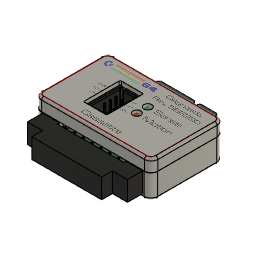
Diag_CP_PCB_v1 v16 (Autodesk Fusion 360 design; units mm, degrees)
Autodesk Fusion 360 part; units mm, degrees
note: some values were not read from the file. Chosen so that the rebuilt part matches the saved one: which bodies a step acts on; which face or edge a step refers to.
sketch "dxf import" plane through (0, 0, 0) normal (0, 0, 1) x (1, 0, 0) in component "PCB"
  line L0 (29, 0) -> (1, 0)
  line L1 (0.7, 29) -> (0, 29)
  line L2 (0, 1) -> (0, 29)
  arc A0 (0.7, 29) -> (1.5, 29.8) centre (0.7, 29.8) ccw
  arc A1 (28.5, 30.8) -> (29.3, 30) centre (29.3, 30.8) ccw
  line L3 (30, 30) -> (30, 29)
  line L4 (29.3, 30) -> (30, 30)
  line L5 (30, 29) -> (30, 1)
  line L6 (1.5, 31) -> (1.5, 29.8)
  line L7 (26, 43) -> (27.5, 43)
  line L8 (27.5, 43) -> (28.5, 42)
  line L9 (28.5, 42) -> (28.5, 31)
  line L10 (1.5, 42) -> (1.5, 31)
  arc A2 (29, 0) -> (30, 1) centre (29, 1) ccw
  line L11 (18.16, 33) -> (18.16, 42.2)
  arc A3 (20.56, 43) -> (19.76, 42.2) centre (20.56, 42.2) ccw
  line L12 (19.76, 42.2) -> (19.76, 33)
  line L13 (28.5, 31) -> (28.5, 30.8)
  arc A4 (0, 1) -> (1, 0) centre (1, 1) ccw
  line L14 (17.36, 43) -> (2.5, 43)
  arc A5 (18.16, 33) -> (18.96, 32.2) centre (18.96, 33) ccw
  line L15 (2.5, 43) -> (1.5, 42)
  line L16 (26, 43) -> (20.56, 43)
  arc A6 (18.96, 32.2) -> (19.76, 33) centre (18.96, 33) ccw
  arc A7 (18.16, 42.2) -> (17.36, 43) centre (17.36, 42.2) ccw
  line L17 (14.72, 0) -> (14.72, -1)
  line L18 (22.64, 0) -> (22.64, -1)
  line L19 (15.95, 0.1) -> (15.95, -1)
  line L20 (17.95, 0.1) -> (17.95, -1)
  line L21 (21.91, 0.1) -> (21.91, -1)
  line L22 (27.1, 0) -> (26.6, 0)
  line L23 (19.18, 0) -> (18.68, 0)
  line L24 (15.22, 0) -> (14.72, 0)
  circle A8 centre (25.4, 25.4) radius 1.7463
  line L25 (23.14, 0) -> (22.64, 0)
  line L26 (10.76, 0) -> (10.76, -1)
  line L27 (25.87, 0.1) -> (25.87, -1)
  line L28 (15.22, -1) -> (15.22, 0)
  circle A9 centre (25.4, 25.4) radius 3.1789
  line L29 (11.26, -1) -> (11.26, 0)
  line L30 (23.14, -1) -> (23.14, 0)
  line L31 (18.68, 0) -> (18.68, -1)
  line L32 (26.6, 0) -> (26.6, -1)
  line L33 (19.18, -1) -> (19.18, 0)
  line L34 (13.99, 0.1) -> (13.99, -1)
  line L35 (23.87, 0.1) -> (23.87, -1)
  line L36 (19.91, 0.1) -> (19.91, -1)
  line L37 (27.1, -1) -> (27.1, 0)
  line L38 (11.99, 0.1) -> (11.99, -1)
  line L39 (11.26, 0) -> (10.76, 0)
  line L40 (-4.15, -8.7333) -> (-4.15, -11.6)
  line L41 (0.05, -1) -> (0.05, 0)
  line L42 (34.09, -11.6) -> (34.09, -8.7333)
  line L43 (34.09, -3.6853) -> (34.09, -3.548)
  line L44 (-5.85, -6.8) -> (-5.85, -5.2)
  line L45 (10.03, 0.1) -> (10.03, -1)
  line L46 (37.34, -6.8) -> (35.79, -6.8)
  line L47 (34.09, -8.052) -> (34.09, -7.9147)
  line L48 (-5.85, -1.6) -> (-5.85, 0)
  line L49 (-4.15, 0) -> (-4.15, -2.8667)
  line L50 (-5.85, -6.8) -> (-7.4, -6.8)
  line L51 (35.79, 0) -> (34.09, 0)
  line L52 (8.03, 0.1) -> (8.03, -1)
  line L53 (37.34, 0) -> (35.79, 0)
  line L54 (3.34, -1) -> (3.34, 0)
  line L55 (34.09, -7.2333) -> (34.09, -4.3667)
  line L56 (-2.45, -6.8) -> (-5.85, -6.8)
  line L57 (-5.85, -4.2) -> (-5.85, -2.6)
  line L58 (-2.45, 0) -> (-4.15, 0)
  line L59 (32.39, -6.8) -> (30.59, -6.8)
  line L60 (0.05, 0) -> (-2.45, 0)
  line L61 (34.09, -2.8667) -> (34.09, 0)
  line L62 (-2.45, -6.8) -> (-2.45, -5.2)
  line L63 (-5.85, 0) -> (-7.4, 0)
  line L64 (-2.45, -1.6) -> (-2.45, 0)
  line L65 (-2.45, -4.2) -> (-2.45, -2.6)
  line L66 (-0.65, -11.6) -> (-0.65, -6.8)
  line L67 (32.39, 0) -> (29.89, 0)
  line L68 (-7.4, 0) -> (-7.4, -6.8)
  line L69 (30.59, -11.6) -> (-0.65, -11.6)
  line L70 (7.3, 0) -> (6.8, 0)
  line L71 (-0.65, -6.8) -> (-2.45, -6.8)
  line L72 (1.4287, 6.0325) -> (2.6987, 6.0325)
  line L73 (3.3338, 5.3975) -> (3.3338, 4.1275)
  line L74 (2.6987, 6.0325) -> (3.3338, 5.3975)
  line L75 (30.59, -6.8) -> (30.59, -11.6)
  line L76 (37.34, 0) -> (37.34, -6.8)
  line L77 (16.0338, 11.43) -> (16.0338, 8.89)
  line L78 (23.6538, 11.43) -> (16.0338, 11.43)
  line L79 (6.8, 0) -> (6.8, -1)
  line L80 (0.7938, 4.1275) -> (0.7938, 5.3975)
  line L81 (0.7938, 5.3975) -> (1.4287, 6.0325)
  line L82 (16.8275, 24.4475) -> (16.8275, 26.9875)
  line L83 (4.07, 0.1) -> (4.07, -1)
  line L84 (34.09, 0) -> (32.39, 0)
  line L85 (6.07, 0.1) -> (6.07, -1)
  line L86 (1.4287, 3.4925) -> (2.6987, 3.4925)
  line L87 (-4.15, -7.9147) -> (-4.15, -8.052)
  line L88 (-4.15, -3.548) -> (-4.15, -3.6853)
  line L89 (2.6987, 3.4925) -> (3.3338, 4.1275)
  line L90 (0.7938, 4.1275) -> (1.4287, 3.4925)
  line L91 (16.0338, 10.16) -> (15.2718, 10.16)
  line L92 (7.3, -1) -> (7.3, 0)
  line L93 (3.34, 0) -> (2.84, 0)
  line L94 (-4.15, 0) -> (-5.85, 0)
  arc A10 (25.5672, 18.0901) -> (21.3677, 19.3984) centre (23.0187, 17.3038) ccw
  line L95 (-4.15, -4.3667) -> (-4.15, -7.2333)
  line L96 (15.875, 22.3838) -> (13.335, 22.3838)
  line L97 (9.2075, 24.4475) -> (16.8275, 24.4475)
  line L98 (29.89, 0) -> (29.89, -1)
  line L99 (15.875, 14.7637) -> (15.875, 22.3838)
  line L100 (35.79, -4.2) -> (35.79, -2.6)
  line L101 (23.6538, 10.16) -> (24.4158, 10.16)
  line L102 (16.8275, 25.7175) -> (17.5895, 25.7175)
  line L103 (35.79, -6.8) -> (32.39, -6.8)
  line L104 (29.89, -1) -> (0.05, -1)
  line L105 (35.79, -6.8) -> (35.79, -5.2)
  line L106 (2.84, 0) -> (2.84, -1)
  arc A11 (17.8675, 14.44) -> (20.8675, 14.44) centre (19.3675, 15.24) ccw
  line L107 (14.605, 14.7637) -> (14.605, 14.0018)
  line L108 (21.3678, 19.3987) -> (21.3678, 15.2088)
  line L109 (16.0338, 8.89) -> (23.6538, 8.89)
  line L110 (13.335, 14.7637) -> (15.875, 14.7637)
  arc A12 (20.8675, 16.04) -> (17.8675, 16.04) centre (19.3675, 15.24) ccw
  line L111 (13.335, 22.3838) -> (13.335, 14.7637)
  arc A13 (21.3677, 15.2087) -> (25.5672, 16.5169) centre (23.0187, 17.3032) ccw
  line L112 (22.7647, 19.9588) -> (22.7647, 19.5578)
  line L113 (16.8275, 26.9875) -> (9.2075, 26.9875)
  line L114 (9.2075, 25.7175) -> (8.4455, 25.7175)
  arc A14 (20.8675, 16.04) -> (17.8675, 16.04) centre (19.3675, 15.24) ccw
  line L115 (22.7647, 15.0498) -> (22.7647, 14.6488)
  arc A15 (17.8675, 14.44) -> (20.8675, 14.44) centre (19.3675, 15.24) ccw
  line L116 (23.6538, 8.89) -> (23.6538, 11.43)
  line L117 (14.605, 22.3838) -> (14.605, 23.1457)
  line L118 (22.7647, 17.5898) -> (22.7647, 17.0177)
  line L119 (9.2075, 26.9875) -> (9.2075, 24.4475)
  line L120 (4.33, 9.1737) -> (4.8062, 9.65)
  arc A16 (3.5362, 10.92) -> (3.5362, 9.65) centre (3.5362, 10.285) ccw
  line L121 (11.95, 9.1737) -> (11.4738, 9.65)
  arc A17 (3.5362, 16.4763) -> (3.5362, 15.3651) centre (3.5362, 15.9207) ccw
  line L122 (6.3937, 23.62) -> (12.7438, 23.62)
  line L123 (4.33, 9.1737) -> (4.965, 9.1737)
  arc A18 (3.5362, 22.35) -> (3.5362, 21.08) centre (3.5362, 21.715) ccw
  line L124 (4.33, 9.1737) -> (4.33, 22.8263)
  line L125 (11.4738, 22.35) -> (11.4738, 17.27)
  line L126 (6.3937, 22.35) -> (11.4738, 22.35)
  line L127 (12.7438, 8.38) -> (6.3937, 8.38)
  line L128 (6.3937, 9.65) -> (6.3937, 9.1737)
  line L129 (4.965, 9.1737) -> (4.965, 8.38)
  line L130 (4.965, 9.65) -> (4.965, 9.1737)
  line L131 (6.3937, 9.1737) -> (11.95, 9.1737)
  line L132 (3.5362, 23.62) -> (4.965, 23.62)
  line L133 (11.95, 14.73) -> (11.95, 9.1737)
  line L134 (4.965, 22.8263) -> (4.33, 22.8263)
  line L135 (6.3937, 9.65) -> (4.965, 9.65)
  line L136 (12.7438, 14.73) -> (12.7438, 8.38)
  line L137 (4.8062, 22.35) -> (4.965, 22.35)
  line L138 (4.965, 22.35) -> (4.965, 22.8263)
  line L139 (3.5362, 8.38) -> (3.5362, 23.62)
  line L140 (6.3937, 8.38) -> (4.965, 8.38)
  line L141 (4.8062, 9.65) -> (4.8062, 22.35)
  line L142 (11.4738, 14.73) -> (11.4738, 9.65)
  line L143 (6.3937, 9.1737) -> (6.3937, 8.38)
  line L144 (4.965, 22.35) -> (6.3937, 22.35)
  line L145 (11.4738, 14.73) -> (11.95, 14.73)
  line L146 (11.4738, 17.27) -> (11.4738, 14.73)
  line L147 (11.95, 14.73) -> (12.7438, 14.73)
  line L148 (4.965, 22.8263) -> (4.965, 23.62)
  line L149 (4.965, 8.38) -> (3.5362, 8.38)
  line L150 (11.4738, 17.27) -> (11.95, 17.27)
  line L151 (4.965, 23.62) -> (6.3937, 23.62)
  line L152 (11.95, 17.27) -> (11.95, 22.8263)
  line L153 (6.3937, 22.35) -> (6.3937, 22.8263)
  line L154 (6.3937, 22.8263) -> (6.3937, 23.62)
  line L155 (6.3937, 22.8263) -> (11.95, 22.8263)
  line L156 (12.7438, 23.62) -> (12.7438, 17.27)
  line L157 (12.7438, 17.27) -> (12.7438, 14.73)
  line L158 (11.95, 17.27) -> (12.7438, 17.27)
  line L159 (11.4738, 9.65) -> (6.3937, 9.65)
  line L160 (4.965, 9.65) -> (4.8062, 9.65)
  line L161 (35.79, -1.6) -> (35.79, 0)
  line L162 (32.39, -1.6) -> (32.39, 0)
  line L163 (4.8062, 22.35) -> (4.33, 22.8263)
  line L164 (32.39, -4.2) -> (32.39, -2.6)
  line L165 (32.39, -6.8) -> (32.39, -5.2)
  line L166 (11.4738, 22.35) -> (11.95, 22.8263)
  line L167 (11.99, 0.1) -> (11.99, 4)
  line L168 (13.99, 0.1) -> (13.99, 4)
  arc A19 (13.99, 4) -> (11.99, 4) centre (12.99, 4) ccw
  arc A20 (25.87, 4) -> (23.87, 4) centre (24.87, 4) ccw
  line L169 (23.87, 0.1) -> (23.87, 4)
  arc A21 (16.45, 2) -> (17.45, 2) centre (16.95, 2) ccw
  arc A22 (17.45, 3) -> (16.45, 3) centre (16.95, 3) ccw
  arc A23 (20.41, 2) -> (21.41, 2) centre (20.91, 2) ccw
  line L170 (19.91, 0.1) -> (19.91, 4)
  line L171 (13.49, 3) -> (13.49, 2)
  line L172 (12.49, 3) -> (12.49, 2)
  arc A24 (13.49, 3) -> (12.49, 3) centre (12.99, 3) ccw
  arc A25 (12.49, 2) -> (13.49, 2) centre (12.99, 2) ccw
  line L173 (25.37, 3) -> (25.37, 2)
  line L174 (20.41, 3) -> (20.41, 2)
  line L175 (17.45, 3) -> (17.45, 2)
  arc A26 (21.41, 3) -> (20.41, 3) centre (20.91, 3) ccw
  arc A27 (25.37, 3) -> (24.37, 3) centre (24.87, 3) ccw
  line L176 (17.95, 0.1) -> (17.95, 4)
  line L177 (16.45, 3) -> (16.45, 2)
  line L178 (21.41, 3) -> (21.41, 2)
  line L179 (5.57, 3) -> (5.57, 2)
  arc A28 (9.53, 3) -> (8.53, 3) centre (9.03, 3) ccw
  arc A29 (8.53, 2) -> (9.53, 2) centre (9.03, 2) ccw
  line L180 (6.616, 13.714) -> (6.616, 13.206)
  line L181 (9.664, 13.206) -> (9.664, 13.714)
  line L182 (7.124, 18.794) -> (6.616, 18.794)
  line L183 (6.616, 15.746) -> (7.124, 15.746)
  line L184 (7.124, 13.206) -> (7.124, 13.714)
  line L185 (24.37, 3) -> (24.37, 2)
  line L186 (7.124, 16.254) -> (6.616, 16.254)
  line L187 (6.616, 16.254) -> (6.616, 15.746)
  line L188 (9.156, 15.746) -> (9.664, 15.746)
  line L189 (1.8098, 5.0165) -> (1.8098, 4.5085)
  line L190 (8.53, 3) -> (8.53, 2)
  line L191 (2.3178, 5.0165) -> (1.8098, 5.0165)
  line L192 (9.156, 13.714) -> (9.156, 13.206)
  arc A30 (5.57, 3) -> (4.57, 3) centre (5.07, 3) ccw
  line L193 (4.07, 0.1) -> (4.07, 4)
  line L194 (10.03, 0.1) -> (10.03, 4)
  arc A31 (17.95, 4) -> (15.95, 4) centre (16.95, 4) ccw
  line L195 (4.57, 3) -> (4.57, 2)
  line L196 (15.95, 0.1) -> (15.95, 4)
  arc A32 (10.03, 4) -> (8.03, 4) centre (9.03, 4) ccw
  line L197 (7.124, 15.746) -> (7.124, 16.254)
  line L198 (6.616, 18.286) -> (7.124, 18.286)
  line L199 (9.664, 13.714) -> (9.156, 13.714)
  line L200 (9.156, 18.286) -> (9.664, 18.286)
  line L201 (7.124, 13.714) -> (6.616, 13.714)
  line L202 (9.156, 18.794) -> (9.156, 18.286)
  line L203 (7.124, 18.286) -> (7.124, 18.794)
  line L204 (21.91, 0.1) -> (21.91, 4)
  arc A33 (24.37, 2) -> (25.37, 2) centre (24.87, 2) ccw
  line L205 (9.53, 3) -> (9.53, 2)
  line L206 (9.156, 13.206) -> (9.664, 13.206)
  line L207 (9.664, 18.794) -> (9.156, 18.794)
  line L208 (2.3178, 4.5085) -> (2.3178, 5.0165)
  line L209 (9.156, 16.254) -> (9.156, 15.746)
  arc A34 (6.07, 4) -> (4.07, 4) centre (5.07, 4) ccw
  arc A35 (4.57, 2) -> (5.57, 2) centre (5.07, 2) ccw
  line L210 (6.07, 0.1) -> (6.07, 4)
  line L211 (9.664, 15.746) -> (9.664, 16.254)
  line L212 (6.616, 18.794) -> (6.616, 18.286)
  arc A36 (21.91, 4) -> (19.91, 4) centre (20.91, 4) ccw
  line L213 (8.03, 0.1) -> (8.03, 4)
  line L214 (9.664, 16.254) -> (9.156, 16.254)
  line L215 (6.616, 13.206) -> (7.124, 13.206)
  line L216 (20.8675, 16.04) -> (20.8675, 14.44)
  circle A37 centre (19.3675, 15.24) radius 1.5
  arc A38 (17.8675, 16.04) -> (17.8675, 14.44) centre (19.3675, 15.24) ccw
  circle A39 centre (19.3675, 20.1613) radius 1.5
  line L217 (9.664, 18.286) -> (9.664, 18.794)
  line L218 (1.8098, 4.5085) -> (2.3178, 4.5085)
  arc A40 (25.5673, 16.5175) -> (25.5673, 18.0901) centre (23.0188, 17.3038) ccw
  line L219 (22.7647, 19.5578) -> (22.7647, 17.5898)
  line L220 (22.7647, 17.0177) -> (22.7647, 15.0498)
  line L221 (25.87, 0.1) -> (25.87, 4)
  line L222 (20.8588, 20.9774) -> (20.876, 19.3775)
  arc A41 (20.8588, 20.9774) -> (20.876, 19.3775) centre (19.3675, 20.1613) ccw
  line L223 (1.8098, 5.0165) -> (2.3178, 4.5085) construction
  constraint tangent A39 L222
extrude "Extrude1" add sketch "dxf import" against normal blind 1.6 contours L0 L1 L2 A0 A1 L3 L4 L5 L6 L7 L8 L9 L10 A2 L11 A3 L12 L13 A4 L14 A5 L15 L16 A6 A7 L19 L20 L21 L22 L23 L24 L25 L27 L34 L35 L36 L38 L39 L45 L52 L70 L83 L85 L93 L167 L168 A19 A20 L169 L170 L176 L193 L194 A31 L196 A32 L204 A34 L210 A36 L213 L221 | L0 L27 L35 A20 L169 L221 | L0 L21 L36 L170 L204 A36 | L0 L19 L20 L176 A31 L196 | L0 L34 L38 L167 L168 A19 | L0 L45 L52 L194 A32 L213 | L0 L83 L85 L193 A34 L210 | A9 | L72 L73 L74 L80 L81 L86 L89 L90 | L77 L78 L109 L116 | L82 L97 L113 L119 | A10 A13 L112 L115 L118 A40 L219 L220 | A10 L108 A13 L112 L115 L118 L219 L220 | L96 L99 L110 L111 | A37 | A11 A12 A14 A15 L216 A38 | L120 L124 L141 L163 | L120 L123 L130 L160 | L123 L124 L129 L132 L134 L139 L148 L149 | L125 L126 L135 L137 L141 L142 L144 L146 L159 L160 | L128 L129 L130 L135 L140 L143 | L134 L137 L138 L163 | L138 L144 L148 L151 L153 L154 | L121 L128 L131 L159 | L127 L131 L133 L136 L143 L147 | L126 L153 L155 L166 | L121 L133 L142 L145 | A16 L139 | L122 L152 L154 L155 L156 L158 | L125 L150 L152 L166 | L145 L146 L147 L150 L157 L158 | A18 L139 | A17 L139 | A21 A22 L175 L177 | A23 L174 A26 L178 | L171 L172 A24 A25 | L173 A27 L185 A33 | L179 A30 L195 A35 | A28 A29 L190 L205 | L180 L184 L201 L215 | L181 L192 L199 L206 | L182 L198 L203 L212 | L183 L186 L187 L197 | L188 L209 L211 L214 | L189 L191 L208 L218 | L200 L202 L207 L217 | A39 | L222 A41 makes body 1 in component "PCB"
extrude "Extrude2" add sketch "dxf import" along normal blind 2.2 contours L125 L126 L135 L137 L141 L142 L144 L146 L159 L160 | L128 L129 L130 L135 L140 L143 | L138 L144 L148 L151 L153 L154 | L145 L146 L147 L150 L157 L158 bodies 1 in component "PCB"
extrude "Extrude3" add sketch "dxf import" along normal blind 8.5 contours L180 L184 L201 L215 | L181 L192 L199 L206 | L182 L198 L203 L212 | L183 L186 L187 L197 | L188 L209 L211 L214 | L200 L202 L207 L217 bodies 1 in component "PCB"
extrude "Extrude4" add sketch "dxf import" along normal blind 8.8 contours L120 L124 L141 L163 | L120 L123 L130 L160 | L123 L124 L129 L132 L134 L139 L148 L149 | L134 L137 L138 L163 | L121 L128 L131 L159 | L127 L131 L133 L136 L143 L147 | L126 L153 L155 L166 | L121 L133 L142 L145 | L122 L152 L154 L155 L156 L158 | L125 L150 L152 L166 bodies 1 in component "PCB"
chamfer "Chamfer1" distance 0.5 angle 45 7 edges at (4.8062, 16, 8.8) (4.8856, 9.65, 8.8) (4.8856, 22.35, 8.8) (8.9337, 9.65, 8.8) (11.4738, 12.19, 8.8) (11.4738, 19.81, 8.8) (8.9337, 22.35, 8.8) on bodies 1 in component "PCB"
extrude "Extrude5" add sketch "dxf import" along normal blind 4.4 from surface at 5.5 separate body contours A37 | A39 makes body 2 at (17.875, 20.0119, 8.4333) makes body 3 at (20.8656, 15.1652, 8.4333) in component "PCB"
extrude "Extrude6" add sketch "dxf import" along normal blind 1 from surface at 5.5 contours A11 A12 A14 A15 L216 A38 bodies 3 in component "PCB"
extrude "Extrude7" add sketch "dxf import" along normal blind 1 from surface at 5.5 contours L222 A41 bodies 2 in component "PCB"
fillet "Fillet1" radius 1.45 2 edges at (17.969, 19.6189, 9.9) (17.969, 14.6976, 9.9) on bodies 2 3 in component "PCB"
extrude "Extrude8" add sketch "dxf import" along normal blind 8.8 from surface at -4.6 separate body contours L0 L22 L32 L37 L104 | L41 L46 L50 L51 L53 L56 L58 L59 L60 L63 L66 L67 L68 L69 L71 L75 L76 L84 L94 L98 L103 L104 | L0 L18 L25 L30 L104 | L0 L23 L31 L33 L104 | L0 L17 L24 L28 L104 | L0 L26 L29 L39 L104 | L0 L70 L79 L92 L104 | L0 L54 L93 L104 L106 makes body 4 in component "PCB"
extrude "Extrude9" add sketch "dxf import" against normal blind 0.5 from surface at -1.6 contours L0 L27 L35 L104 | L0 L27 L35 A20 L169 L221 | L0 L21 L36 L104 | L0 L21 L36 L170 L204 A36 | L0 L19 L20 L104 | L0 L19 L20 L176 A31 L196 | L0 L34 L38 L104 | L0 L34 L38 L167 L168 A19 | L0 L45 L52 L104 | L0 L45 L52 L194 A32 L213 | L0 L83 L85 L104 | L0 L83 L85 L193 A34 L210 bodies 1 4 in component "PCB"
combine "Combine1" operation add target body 1 tool bodies 2 3 makes body 5 at (17.875, 20.0119, 7.8) makes body 6 at (20.86, 15.0906, 7.15) in component "PCB"
combine "Combine2" operation add target body 1 tool bodies 5 6 makes body 7 at (17.875, 20.0119, 7.8) makes body 8 at (20.86, 15.0906, 7.15) in component "PCB"
ref_plane "WorkPlane1" through (0, 0, -4.4) normal (0, 0, 1) x (1, 0, 0) in component "diag cp bottom shell"
sketch "bottom shell" plane through (0, 0, -4.4) normal (0, 0, 1) x (1, 0, 0) in component "diag cp bottom shell"
  line L0 (30, 30) -> (30, 1) construction
  line L1 (0, 1) -> (0, 29) construction
  line L2 (2.84, 0) -> (1, 0) construction
  circle A0 centre (25.4, 25.4) radius 1.7463 construction
  line L3 (-11, 3) -> (-11, 29.5)
  line L4 (-8, 32.5) -> (38, 32.5)
  line L5 (38, 0) -> (-8, 0)
  line L6 (41, 29.5) -> (41, 3)
  arc A1 (-8, 32.5) -> (-11, 29.5) centre (-8, 29.5) ccw
  arc A2 (41, 29.5) -> (38, 32.5) centre (38, 29.5) ccw
  arc A3 (38, 0) -> (41, 3) centre (38, 3) ccw
  arc A4 (-11, 3) -> (-8, 0) centre (-8, 3) ccw
  circle A5 centre (25.4, 25.4) radius 1.75
  circle A6 centre (25.4, 25.4) radius 3
  circle A7 centre (25.4, 25.4) radius 4.25
  arc A8 (39, 29.5) -> (38, 30.5) centre (38, 29.5) ccw
  line L7 (-8, 30.5) -> (38, 30.5)
  arc A9 (-8, 30.5) -> (-9, 29.5) centre (-8, 29.5) ccw
  line L8 (-9, 3) -> (-9, 29.5)
  arc A10 (-9, 3) -> (-8, 2) centre (-8, 3) ccw
  line L9 (38, 2) -> (-8, 2)
  arc A11 (38, 2) -> (39, 3) centre (38, 3) ccw
  line L10 (39, 29.5) -> (39, 3)
  arc A12 (39.8, 29.5) -> (38, 31.3) centre (38, 29.5) ccw
  arc A13 (-8, 31.3) -> (-9.8, 29.5) centre (-8, 29.5) ccw
  line L11 (-9.8, 3) -> (-9.8, 29.5)
  arc A14 (-9.8, 3) -> (-8, 1.2) centre (-8, 3) ccw
  arc A15 (38, 1.2) -> (39.8, 3) centre (38, 3) ccw
  line L12 (39.8, 29.5) -> (39.8, 3)
  line L13 (30.3, 2) -> (30.3, 0)
  line L14 (-0.3, 2) -> (-0.3, 0)
  line L15 (1.5, 42) -> (1.5, 29.8) construction
  line L16 (28.5, 42) -> (28.5, 30.8) construction
  line L17 (28.8, 32.5) -> (28.8, 30.5)
  line L18 (1.2, 32.5) -> (1.2, 30.5)
  line L19 (-8, 31.3) -> (1.5, 31.3)
  line L20 (28.5, 31.3) -> (38, 31.3)
  line L21 (38, 1.2) -> (30, 1.2)
  line L22 (0, 1.2) -> (-8, 1.2)
  circle A16 centre (-4.5, 6.5) radius 1.75
  circle A17 centre (34.5, 6.5) radius 1.75
  circle A18 centre (-4.5, 6.5) radius 4
  circle A19 centre (34.5, 6.5) radius 4
  circle A20 centre (-4.5, 6.5) radius 3
  circle A21 centre (34.5, 6.5) radius 3
  line L23 (25.4, 25.4) -> (-9, 25.4) construction
  line L24 (-2, 26.4) -> (2, 26.4)
  line L25 (2, 26.4) -> (2, 24.4)
  line L26 (2, 24.4) -> (-2, 24.4)
  line L27 (-2, 24.4) -> (-2, 26.4)
  line L28 (-0.3, 26.4) -> (-0.3, 24.4)
  point P0 (-11, 0)
  point P1 (-11, 32.5)
  point P2 (41, 32.5)
  dimension "d54" = 3
  dimension "d55" = 11
  dimension "d56" = 32.5
  dimension "d57" = 52
  dimension "d59" = 3.5
  dimension "d63" = 6
  dimension "d64" = 8.5
  dimension "d65" = 2
  dimension "d68" = 0.3
  dimension "d69" = 0.3
  dimension "d70" = 0.3
  dimension "d71" = 0.3
  dimension "d72" = 1.2
  dimension "d73" = 3.5
  dimension "d74" = 4.5
  dimension "d75" = 4.5
  dimension "d76" = 3.5
  dimension "d77" = 4.5
  dimension "d78" = 4.5
  dimension "d80" = 8
  dimension "d81" = 8
  dimension "d82" = 6
  dimension "d83" = 6
  dimension "d84" = 4
  dimension "d85" = 2
  dimension "d86" = 0.3
  constraint parallel L1 L3
  constraint perpendicular L1 L4
  constraint perpendicular L1 L5
  constraint coincident L2.start L5
  constraint perpendicular L5 L6
  constraint coincident P1 L3
  constraint coincident P1 L4
  constraint tangent L3 A1
  constraint tangent L4 A1
  constraint coincident P2 L4
  constraint coincident P2 L6
  constraint tangent L4 A2
  constraint tangent L6 A2
  constraint equal A1 A2
  constraint tangent L6 A3
  constraint tangent L5 A3
  constraint equal A1 A3
  constraint coincident P0 L3
  constraint coincident P0 L5
  constraint tangent L3 A4
  constraint tangent L5 A4
  constraint equal A1 A4
  constraint concentric A0 A5
  constraint concentric A5 A6
  constraint concentric A6 A7
  constraint coincident L9 L13.start
  constraint coincident L5 L13.end
  constraint perpendicular L5 L13
  constraint coincident L9 L14.start
  constraint coincident L5 L14.end
  constraint perpendicular L5 L14
  constraint coincident L4 L17.start
  constraint coincident L7 L17.end
  constraint perpendicular L7 L17
  constraint coincident L4 L18.start
  constraint coincident L7 L18.end
  constraint perpendicular L7 L18
  constraint concentric A2 A12
  constraint parallel L4 L19
  constraint concentric A1 A13
  constraint parallel L3 L11
  constraint concentric A4 A14
  constraint parallel L5 L21
  constraint concentric A3 A15
  constraint parallel L6 L12
  constraint tangent A13 L19
  constraint tangent A12 L12
  constraint tangent A12 L19
  constraint tangent A13 L11
  constraint tangent L11 A14
  constraint tangent A14 L21
  constraint tangent A15 L21
  constraint tangent A15 L12
  constraint coincident L15 L19.end
  constraint coincident L16 L20.start
  constraint collinear L19 L20
  constraint coincident L0 L21.end
  constraint coincident L1 L22.start
  constraint collinear L21 L22
  constraint concentric A16 A18
  constraint concentric A17 A19
  constraint concentric A16 A20
  constraint concentric A19 A21
  constraint coincident A0.centre A5.centre
  constraint coincident L8 L23.end
  constraint perpendicular L8 L23
  constraint horizontal L24
  constraint vertical L25
  constraint horizontal L26
  constraint vertical L27
  constraint symmetric L23 L24 L26
  constraint symmetric L1 L25 L27
  constraint coincident L24 L28.start
  constraint coincident L26 L28.end
  constraint perpendicular L26 L28
  measures "d54" radius of A1
  measures "d55" distance of L1 L3
  measures "d56" distance of L4 L5
  measures "d57" distance of L3 L6
  measures "d59" diameter of A5
  measures "d63" diameter of A6
  measures "d64" diameter of A7
  measures "d68" distance of L1 L14
  measures "d69" distance of L0 L13
  measures "d70" distance of L16 L17
  measures "d71" distance of L15 L18
  measures "d72" distance of L6 L12
  measures "d73" diameter of A16
  measures "d74" distance of L1 A16.centre
  measures "d75" distance of L9 A16.centre
  measures "d76" diameter of A17
  measures "d77" distance of L0 A17.centre
  measures "d78" distance of L9 A17.centre
  measures "d80" diameter of A18
  measures "d81" diameter of A19
  measures "d82" diameter of A20
  measures "d83" diameter of A21
  measures "d84" distance of L25 L27
  measures "d85" distance of L24 L26
  measures "d86" distance of L1 L28
extrude "Extrude1'" add sketch "bottom shell" against normal blind 2 separate body contours L3 L4 L5 A1 A4 A13 L11 A14 L14 L18 L19 L22 | L5 L9 L13 L14 | L4 L7 L17 L18 | L4 L5 L6 A2 A3 A12 A15 L12 L13 L17 L20 L21 | L7 A9 L8 A10 L9 A13 L11 A14 L14 L18 L19 L22 | A8 L7 L9 A11 L10 A12 A15 L12 L13 L17 L20 L21 | A8 L7 A9 L8 A10 L9 A11 L10 | A7 | A18 | A19 | L24 L26 L27 L28 | L24 L25 L26 L28 makes body 9 in component "diag cp bottom shell"
extrude "Extrude2'" add sketch "bottom shell" along normal blind 2.8 contours A6 | A7 | L24 L25 L26 L28 bodies 9 in component "diag cp bottom shell"
extrude "Extrude3'" add sketch "bottom shell" along normal blind 4.4 contours A18 | A19 | A20 | A21 | L24 L26 L27 L28 bodies 9 in component "diag cp bottom shell"
chamfer "Chamfer1'" distance 1.3 angle 45 1 edges at (21.4376, 23.8631, -1.6) on bodies 9 in component "diag cp bottom shell"
extrude "Extrude4'" add sketch "bottom shell" along normal blind 2.8 contours L4 L7 L17 L18 bodies 9 in component "diag cp bottom shell"
extrude "Extrude5'" add sketch "bottom shell" along normal blind 1 contours L5 L9 L13 L14 bodies 9 in component "diag cp bottom shell"
extrude "Extrude6'" add sketch "bottom shell" along normal blind 8.7 contours L3 L4 L5 A1 A4 A13 L11 A14 L14 L18 L19 L22 | L4 L5 L6 A2 A3 A12 A15 L12 L13 L17 L20 L21 bodies 9 in component "diag cp bottom shell"
extrude "Extrude7'" add sketch "bottom shell" along normal blind 9.7 contours L7 A9 L8 A10 L9 A13 L11 A14 L14 L18 L19 L22 | A8 L7 L9 A11 L10 A12 A15 L12 L13 L17 L20 L21 bodies 9 in component "diag cp bottom shell"
fillet "Fillet1'" radius 1 8 edges at (15, 0, -6.4) (-10.1213, 0.8787, -6.4) (-11, 16.25, -6.4) (-10.1213, 31.6213, -6.4) (15, 32.5, -6.4) (40.1213, 31.6213, -6.4) (41, 16.25, -6.4) (40.1213, 0.8787, -6.4) on bodies 9 in component "diag cp bottom shell"
fillet "Fillet2" radius 0.5 8 edges at (15, 2, -4.4) (38.7071, 2.2929, -4.4) (39, 16.25, -4.4) (38.7071, 30.2071, -4.4) (15, 30.5, -4.4) (-8.7071, 30.2071, -4.4) (-9, 16.25, -4.4) (-8.7071, 2.2929, -4.4) on bodies 9 in component "diag cp bottom shell"
fillet "Fillet3" radius 0.5 4 edges at (0, 24.4, -4.4) (2, 25.4, -4.4) (0, 26.4, -4.4) (-2, 25.4, -4.4) on bodies 9 in component "diag cp bottom shell"
fillet "Fillet4" radius 0.5 1 edges at (21.4376, 26.9369, -4.4) on bodies 9 in component "diag cp bottom shell"
fillet "Fillet5" radius 0.5 2 edges at (28.8, 30.5, 1.85) (1.2, 30.5, 1.85) on bodies 9 in component "diag cp bottom shell"
ref_plane "WorkPlane1" through (0, 0, 8) normal (0, 0, 1) x (1, 0, 0) in component "diag cp-top shell"
sketch "top shell" plane through (0, 0, 8) normal (0, 0, 1) x (1, 0, 0) in component "diag cp-top shell"
  line L0 (28.8, 32.5) -> (1.2, 32.5)
  line L1 (0.7, 30.5) -> (29.3, 30.5)
  line L2 (1.2, 32.5) -> (-8, 32.5)
  line L3 (-8, 30.5) -> (0.7, 30.5)
  arc A0 (-8, 32.5) -> (-11, 29.5) centre (-8, 29.5) ccw
  arc A1 (-8, 30.5) -> (-9, 29.5) centre (-8, 29.5) ccw
  line L4 (-11, 29.5) -> (-11, 3)
  line L5 (-9, 3) -> (-9, 29.5)
  arc A2 (-9, 3) -> (-8, 2) centre (-8, 3) ccw
  line L6 (-0.3, 2) -> (-8, 2)
  arc A3 (-11, 3) -> (-8, 0) centre (-8, 3) ccw
  line L7 (-8, 0) -> (-0.3, 0)
  line L8 (30.3, 2) -> (-0.3, 2)
  line L9 (-0.3, 0) -> (30.3, 0)
  line L10 (38, 2) -> (30.3, 2)
  line L11 (30.3, 0) -> (38, 0)
  arc A4 (38, 2) -> (39, 3) centre (38, 3) ccw
  line L12 (39, 29.5) -> (39, 3)
  arc A5 (39, 29.5) -> (38, 30.5) centre (38, 29.5) ccw
  line L13 (29.3, 30.5) -> (38, 30.5)
  line L14 (38, 32.5) -> (28.8, 32.5)
  arc A6 (41, 29.5) -> (38, 32.5) centre (38, 29.5) ccw
  line L15 (41, 3) -> (41, 29.5)
  arc A7 (38, 0) -> (41, 3) centre (38, 3) ccw
  circle A8 centre (25.4, 25.4) radius 1.75 construction
  circle A9 centre (34.5, 6.5) radius 1.75 construction
  circle A10 centre (-4.5, 6.5) radius 1.75 construction
  line L16 (28.5, 42) -> (28.5, 30.8) construction
  line L17 (1.5, 42) -> (1.5, 29.8) construction
  line L18 (30, 30) -> (30, 1) construction
  line L19 (0, 1) -> (0, 29) construction
  line L20 (4.965, 23.62) -> (3.5362, 23.62) construction
  line L21 (3.5362, 23.62) -> (3.5362, 8.38) construction
  line L22 (3.5362, 8.38) -> (4.965, 8.38) construction
  line L23 (6.3937, 8.38) -> (12.7438, 8.38) construction
  line L24 (12.7438, 8.38) -> (12.7438, 14.73) construction
  line L25 (12.7438, 17.27) -> (12.7438, 23.62) construction
  line L26 (12.7438, 23.62) -> (6.3937, 23.62) construction
  circle A11 centre (19.3675, 15.24) radius 1.5 construction
  circle A12 centre (19.3675, 20.1613) radius 1.5 construction
  line L27 (3.4362, 24.22) -> (12.8438, 24.22)
  line L28 (13.3438, 23.72) -> (13.3438, 8.28)
  line L29 (12.8438, 7.78) -> (3.4362, 7.78)
  line L30 (2.9362, 8.28) -> (2.9362, 23.72)
  circle A13 centre (19.3675, 20.1613) radius 1.75
  circle A14 centre (19.3675, 15.24) radius 1.75
  circle A15 centre (25.4, 25.4) radius 1.25
  circle A16 centre (34.5, 6.5) radius 1.25
  circle A17 centre (-4.5, 6.5) radius 1.25
  circle A18 centre (25.4, 25.4) radius 3
  circle A19 centre (34.5, 6.5) radius 3
  circle A20 centre (-4.5, 6.5) radius 3
  line L31 (1.2, 31.7) -> (-8, 31.7)
  arc A21 (-8, 31.7) -> (-10.2, 29.5) centre (-8, 29.5) ccw
  line L32 (-10.2, 29.5) -> (-10.2, 3)
  arc A22 (-10.2, 3) -> (-8, 0.8) centre (-8, 3) ccw
  line L33 (-8, 0.8) -> (-0.3, 0.8)
  line L34 (30.3, 0.8) -> (38, 0.8)
  arc A23 (38, 0.8) -> (40.2, 3) centre (38, 3) ccw
  line L35 (40.2, 3) -> (40.2, 29.5)
  arc A24 (40.2, 29.5) -> (38, 31.7) centre (38, 29.5) ccw
  line L36 (38, 31.7) -> (28.8, 31.7)
  line L37 (1.5, 32.5) -> (1.5, 30.5)
  line L38 (28.5, 32.5) -> (28.5, 30.5)
  line L39 (30, 2) -> (30, 0)
  line L40 (0, 2) -> (0, 0)
  line L41 (28.8, 31.7) -> (28.5, 31.7)
  line L42 (1.5, 31.7) -> (1.2, 31.7)
  line L43 (-0.3, 0.8) -> (0, 0.8)
  line L44 (30, 0.8) -> (30.3, 0.8)
  arc A25 (3.4362, 24.22) -> (2.9362, 23.72) centre (3.4362, 23.72) ccw
  arc A26 (13.3438, 23.72) -> (12.8438, 24.22) centre (12.8438, 23.72) ccw
  arc A27 (12.8438, 7.78) -> (13.3438, 8.28) centre (12.8438, 8.28) ccw
  arc A28 (2.9362, 8.28) -> (3.4362, 7.78) centre (3.4362, 8.28) ccw
  line L45 (1.8098, 5.0165) -> (2.3178, 4.5085)
  circle A29 centre (2.0638, 4.7625) radius 2
  dimension "d110" = 0.6
  dimension "d111" = 0.6
  dimension "d112" = 0.6
  dimension "d113" = 0.6
  dimension "d114" = 3.5
  dimension "d115" = 3.5
  dimension "d116" = 2.5
  dimension "d117" = 2.5
  dimension "d118" = 2.5
  dimension "d119" = 6
  dimension "d120" = 6
  dimension "d121" = 6
  dimension "d123" = 0.8
  dimension "d138" = 0.5
  dimension "d139" = 4
  constraint horizontal L27
  constraint vertical L28
  constraint horizontal L29
  constraint vertical L30
  constraint concentric A12 A13
  constraint concentric A11 A14
  constraint concentric A8 A15
  constraint concentric A9 A16
  constraint concentric A10 A17
  constraint concentric A8 A18
  constraint concentric A16 A19
  constraint concentric A10 A20
  constraint coincident L0 L37.start
  constraint coincident L17 L37.start
  constraint coincident L17 L37.end
  constraint coincident L1 L37.end
  constraint coincident L0 L38.start
  constraint coincident L16 L38.start
  constraint coincident L1 L38.end
  constraint perpendicular L1 L38
  constraint coincident L8 L39.start
  constraint coincident L18 L39.start
  constraint coincident L9 L39.end
  constraint perpendicular L9 L39
  constraint coincident L8 L40.start
  constraint coincident L19 L40.start
  constraint coincident L40.end origin
  constraint parallel L0 L41
  constraint parallel L2 L31
  constraint concentric A0 A21
  constraint parallel L4 L32
  constraint concentric A3 A22
  constraint parallel L7 L33
  constraint parallel L9 L43
  constraint parallel L11 L34
  constraint concentric A7 A23
  constraint parallel L15 L35
  constraint concentric A6 A24
  constraint parallel L14 L36
  constraint tangent A24 L36
  constraint tangent L31 A21
  constraint tangent A21 L32
  constraint tangent L32 A22
  constraint tangent A22 L33
  constraint tangent L34 A23
  constraint tangent L35 A24
  constraint tangent A23 L35
  constraint coincident L16 L41.end
  constraint coincident L17 L42.start
  constraint collinear L41 L42
  constraint coincident L40 L43.end
  constraint coincident L39 L44.start
  constraint collinear L43 L44
  constraint tangent L27 A25
  constraint tangent L30 A25
  constraint tangent L27 A26
  constraint tangent L28 A26
  constraint equal A25 A26
  constraint tangent L28 A27
  constraint tangent L29 A27
  constraint equal A25 A27
  constraint tangent L29 A28
  constraint tangent L30 A28
  constraint equal A25 A28
  constraint midpoint L45 A29.centre
  measures "d110" distance of L26 L27
  measures "d111" distance of L23 L29
  measures "d112" distance of L25 L28
  measures "d113" distance of L21 L30
  measures "d114" diameter of A13
  measures "d115" diameter of A14
  measures "d116" diameter of A15
  measures "d117" diameter of A16
  measures "d118" diameter of A17
  measures "d119" diameter of A18
  measures "d120" diameter of A19
  measures "d121" diameter of A20
  measures "d123" distance of L15 L35
  measures "d138" radius of A25
  measures "d139" diameter of A29
extrude "Extrude1''" add sketch "top shell" along normal blind 2 separate body contours L0 L9 L11 L14 A6 L15 A7 L34 A23 L35 A24 L36 L38 L39 L41 L44 | L0 L1 L37 L38 | L0 L2 A0 L4 A3 L7 L9 L31 A21 L32 A22 L33 L37 L40 L42 L43 | L1 L8 L10 A4 L12 A5 L13 L34 A23 L35 A24 L36 L38 L39 L41 L44 | L1 L3 A1 L5 A2 L6 L8 L31 A21 L32 A22 L33 L37 L40 L42 L43 | L1 L3 A1 L5 A2 L6 L8 L10 A4 L12 A5 L13 | L8 L9 L39 L40 | A15 | A16 | A17 | A18 | A19 | A20 | A29 makes body 10 in component "diag cp-top shell"
extrude "Extrude2''" add sketch "top shell" against normal blind 7.8 contours A18 | A19 | A20 bodies 10 in component "diag cp-top shell"
extrude "Extrude3''" add sketch "top shell" against normal blind 3.5 contours L0 L9 L11 L14 A6 L15 A7 L34 A23 L35 A24 L36 L38 L39 L41 L44 | L0 L2 A0 L4 A3 L7 L9 L31 A21 L32 A22 L33 L37 L40 L42 L43 bodies 10 in component "diag cp-top shell"
extrude "Extrude4''" add sketch "top shell" against normal blind 7.8 contours L0 L1 L37 L38 bodies 10 in component "diag cp-top shell"
extrude "Extrude5''" add sketch "top shell" against normal blind 2.5 separate body contours L1 L8 L10 A4 L12 A5 L13 L34 A23 L35 A24 L36 L38 L39 L41 L44 | L1 L3 A1 L5 A2 L6 L8 L31 A21 L32 A22 L33 L37 L40 L42 L43 makes body 11 at (-10.2, 20.6667, 7.1667) makes body 12 at (40.2, 11.8333, 7.1667) in component "diag cp-top shell"
extrude "Extrude6''" add sketch "top shell" against normal blind 3.5 contours L8 L9 L39 L40 bodies 10 12 11 in component "diag cp-top shell"
fillet "Fillet1''" radius 1 8 edges at (-11, 16.25, 10) (-10.1213, 0.8787, 10) (15, 0, 10) (40.1213, 0.8787, 10) (41, 16.25, 10) (40.1213, 31.6213, 10) (15, 32.5, 10) (-10.1213, 31.6213, 10) on bodies 10 in component "diag cp-top shell"
extrude "Extrude7''" cut sketch "top shell" along normal blind 1.5 contours A29 bodies 10 in component "diag cp-top shell"
fillet "Fillet2'" radius 0.5 1 edges at (0.1991, 4.0393, 9.5) on bodies 10 in component "diag cp-top shell"
fillet "Fillet3'" radius 0.5 3 edges at (-5.6654, 6.952, 8) (33.3346, 6.952, 8) (24.2346, 25.852, 8) on bodies 10 in component "diag cp-top shell"
sketch "Sketch1" plane through (0, 0, 8.5) normal (0, 0, 1) x (-1, 0, 0)
  line L0 (-9.156, -13.206) -> (-9.664, -13.206)
  line L1 (-9.664, -13.206) -> (-9.664, -13.714)
  line L2 (-9.664, -13.714) -> (-9.156, -13.714)
  line L3 (-9.156, -13.714) -> (-9.156, -13.206)
component "PCB" placed x (1, 0, 0) y (0, 1, 0) z (0, 0, 1) at (0, 0, 0)
component "diag cp bottom shell" placed x (1, 0, 0) y (0, 1, 0) z (0, 0, 1) at (0, 0, 0)
component "diag cp-top shell" placed x (1, 0, 0) y (0, 1, 0) z (0, 0, 1) at (0.1348, 0, 0)
equation "below = 2.8 mm + pcb_tickness" comment "inner bottom plane"
equation "width = 48 mm + 2 * wall" comment "width"
equation "wall = 2 mm" comment "wall thickness"
equation "length = 30 mm + 0.5 mm + wall" comment "length"
equation "above = 10 mm - wall" comment "inner top plane"
equation "pcb_tickness = 1.6 mm" comment "pcb thickness"
equation "pcb_width = 30 mm" comment "pcb width"
equation "d49 = -below"
equation "r_corner = 3 mm"
equation "d54 = r_corner"
equation "d55 = ( width - pcb_width ) / 2"
equation "d56 = length"
equation "d57 = width"
equation "drill = 3.5 mm" comment "screw drill"
equation "d_screw = 6 mm" comment "dia screw head"
equation "d_post = 8.5 mm" comment "dia post pcb"
equation "d63 = d_screw"
equation "d64 = d_post"
equation "d65 = wall"
equation "tol_x = 0.3 mm" comment "x gap PCB"
equation "d68 = tol_x"
equation "d69 = tol_x"
equation "d70 = tol_x"
equation "d71 = tol_x"
equation "d72 = wall * 0.6"
equation "d73 = drill"
equation "d74 = ( d55 - wall ) / 2"
equation "d75 = d74"
equation "d76 = drill"
equation "d77 = d74"
equation "d78 = d75"
equation "d_post2 = 8 mm" comment "dia post 2"
equation "d86 = tol_x"
equation "d87 = -wall"
equation "d89 = below - pcb_tickness"
equation "d91 = below"
equation "d94 = below - pcb_tickness"
equation "bottom_height = 4.3 mm + below" comment "top level bottom"
equation "overlap = 1 mm" comment "overlap top bottom shell"
equation "d100 = bottom_height"
equation "d102 = bottom_height + overlap"
equation "d109 = above"
equation "d110 = 2 * tol_x"
equation "d111 = 2 * tol_x"
equation "d112 = 2 * tol_x"
equation "d113 = 2 * tol_x"
equation "d115 = d114"
equation "d119 = d_screw"
equation "d120 = d_screw"
equation "d121 = d_screw"
equation "d123 = wall * 0.4"
equation "d124 = wall"
equation "d126 = -above + tol_y"
equation "d128 = -top_height"
equation "top_height = above + below - bottom_height - tol_y"
equation "d131 = -above + tol_y"
equation "d133 = -top_height + overlap"
equation "d136 = -top_height"
equation "d140 = wall - 0.5 mm"
equation "tol_y = 0.2 mm"
named bodies: "PCB", "ledgn", "ledrd", "bottom shell", "top shell"
